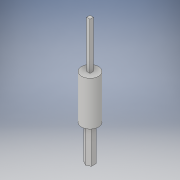
# Autodesk Inventor part: Part1
Saved by Autodesk Inventor 2018 (Build 220112000, 112)
## iProperties
Created: 2018-01-23
Part Number: Part1
Material: Generic
Document SubType Name: Modeling
Designer: prakh
Density: 1 g/cm^3
Appearance: Default
Author: prakh
Autodesk Inventor part; units mm, degrees
ref_plane "YZ Plane" through (0, 0, 0) normal (1, 0, 0) x (0, 1, 0)
ref_plane "XZ Plane" through (0, 0, 0) normal (0, 1, 0) x (-1, 0, 0)
ref_plane "XY Plane" through (0, 0, 0) normal (0, 0, 1) x (1, 0, 0)
sketch "Sketch1" plane through (0, 0, 0) normal (0, 1, 0) x (-1, 0, 0)
  line L0 (0, -4.766) -> (-4.1275, -2.383)
  line L1 (-4.1275, -2.383) -> (-4.1275, 2.383)
  line L2 (-4.1275, 2.383) -> (0, 4.766)
  line L3 (0, 4.766) -> (4.1275, 2.383)
  line L4 (4.1275, 2.383) -> (4.1275, -2.383)
  line L5 (4.1275, -2.383) -> (0, -4.766)
  point P0 (0, 0)
  point P1 (0, 0)
  dimension "d0" = 8.255
  constraints: 12 end point, 1 coincident, 13 other
  measures "d0" distance between parallel lines of L1 L4
extrude "Extrusion1" add sketch "Sketch1" along normal blind 38.1
sketch "Sketch2" plane through (0, 38.1, 0) normal (0, 1, 0) x (1, 0, 0)
  circle A0 centre (0, 0) radius 9.2075
  dimension "d3" = 18.415
  constraints: 1 centre point, 1 coincident
  measures "d3" diameter of A0
extrude "Extrusion2" add sketch "Sketch2" along normal blind 47.625
sketch "Sketch3" plane through (0, 85.725, 0) normal (0, 1, 0) x (1, 0, 0)
  line L0 (-1.8415, 1.8415) -> (1.8415, 1.8415)
  line L1 (1.8415, 1.8415) -> (1.8415, -1.8415)
  line L2 (1.8415, -1.8415) -> (-1.8415, -1.8415)
  line L3 (-1.8415, -1.8415) -> (-1.8415, 1.8415)
  point P0 (0, 0)
  point P1 (0, 0)
  dimension "d6" = 3.683
  constraints: 8 end point, 1 coincident, 9 other
  measures "d6" distance between parallel lines of L1 L3
extrude "Extrusion3" add sketch "Sketch3" along normal blind 50.8
body "Solid1"
